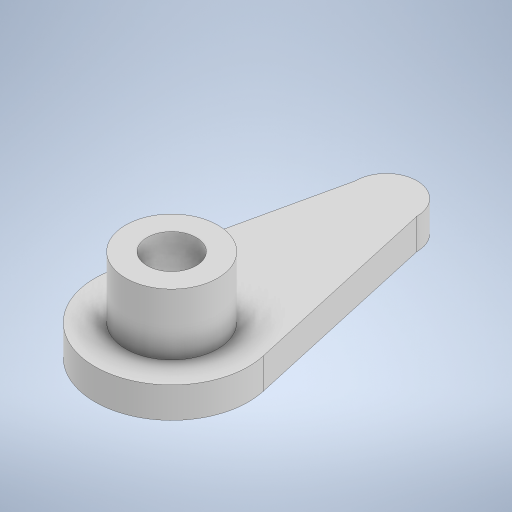
# Autodesk Inventor part: connector1
Saved by Autodesk Inventor 2023 (Build 270158000, 158)
## iProperties
Created: 2022-11-12
Part Number: connector1
Material: Generic
Document SubType Name: Modeling
Designer: forti
Density: 1 g/cm^3
Appearance: Default
Author: forti
Autodesk Inventor part; units mm, degrees
ref_plane "YZ Plane" through (0, 0, 0) normal (1, 0, 0) x (0, 1, 0)
ref_plane "XZ Plane" through (0, 0, 0) normal (0, 1, 0) x (-1, 0, 0)
ref_plane "XY Plane" through (0, 0, 0) normal (0, 0, 1) x (1, 0, 0)
sketch "Sketch1" plane through (0, 0, 0) normal (0, 1, 0) x (-1, 0, 0)
  point P0 (0, 0)
sketch "Sketch2" plane through (0, 0, 0) normal (0, 1, 0) x (-1, 0, 0)
  arc A0 (12.2002, -2.7214) -> (-12.2002, -2.7214) centre (0, 0) ccw
  arc A1 (-5, -35) -> (5, -35) centre (0, -35) ccw
  line L0 (5, -35) -> (12.2002, -2.7214)
  line L1 (-5, -35) -> (-12.2002, -2.7214)
  line L2 (0, 0) -> (0, -12.5)
  line L3 (0, -30) -> (0, -35)
  dimension "d0" = 25
  dimension "d1" = 35
  dimension "d2" = 10
  constraints: 8 end point, 4 point on circle, 2 centre point, 2 coincident, 2 tangent, 2 vertical
  measures "d0" diameter of A0
  measures "d1" distance of L2.start L3.end
  measures "d2" diameter of A1
extrude "Extrusion1" add sketch "Sketch2" along normal blind 5
sketch "Sketch3" plane through (0, 5, 0) normal (0, 1, 0) x (1, 0, 0)
  circle A0 centre (0, 0) radius 4
  circle A1 centre (0, 0) radius 7.5
  dimension "d5" = 8
  dimension "d6" = 15
  constraints: 2 centre point, 2 coincident
  measures "d5" diameter of A0
  measures "d6" diameter of A1
extrude "Extrusion2" add sketch "Sketch3" along normal blind 10
body "Solid1"
